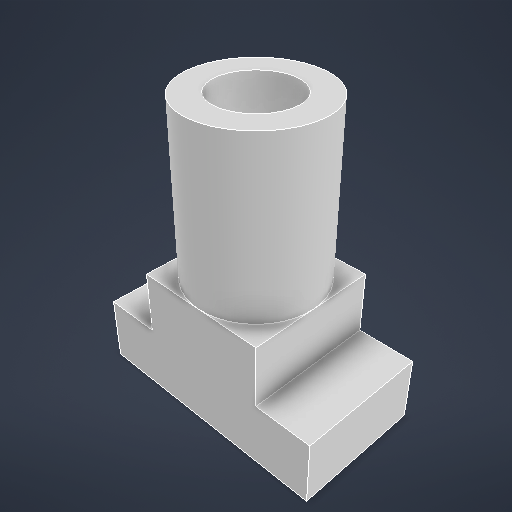
# Autodesk Inventor part: diff_gear_holder_3
Saved by Autodesk Inventor 2025 (Build 290162000, 162)
## iProperties
Created: 2024-07-25
Part Number: diff_gear_holder_3
Material: Generic
Document SubType Name: Modeling
Designer: Garfieldcmix
Density: 1 g/cm^3
Appearance: Default
Author: Garfieldcmix
Autodesk Inventor part; units mm, degrees
ref_plane "YZ Plane" through (0, 0, 0) normal (1, 0, 0) x (0, 1, 0)
ref_plane "XZ Plane" through (0, 0, 0) normal (0, 1, 0) x (-1, 0, 0)
ref_plane "XY Plane" through (0, 0, 0) normal (0, 0, 1) x (1, 0, 0)
sketch "Sketch1" plane through (0, 0, 0) normal (0, 1, 0) x (-1, 0, 0)
  line L0 (0, -8) -> (15, -8)
  line L1 (15, -8) -> (15, 0)
  line L2 (15, 0) -> (0, 0)
  line L3 (0, 0) -> (0, -8)
  line L4 (7.5, 0) -> (7.5, -8) construction
  line L5 (0, -4) -> (15, -4) construction
  line L6 (3.5, 0) -> (3.5, -8)
  line L7 (11.5, -8) -> (11.5, 0)
  circle A0 centre (7.5, -4) radius 2.4
  circle A1 centre (7.5, -4) radius 4
  dimension "d2" = 15
  dimension "d3" = 8
  dimension "d4" = 4
  dimension "d5" = 4
  dimension "d6" = 4.8
  dimension "d7" = 8
  constraints: 16 end point, 5 midpoint, 4 point on line, 3 coincident, 3 perpendicular, 2 centre point, 2 parallel, 1 vertical
  measures "d2" distance of L3.end L0.end
  measures "d3" distance of L2.end L3.end
  measures "d4" distance between parallel lines of L7 L4
  measures "d5" distance between parallel lines of L6 L4
  measures "d6" diameter of A0
  measures "d7" diameter of A1
extrude "Extrusion1" add sketch "Sketch1" along normal blind 4 contours L3 L2 L6 L0 | L7 L2 L1 L0
extrude "Extrusion2" add sketch "Sketch1" along normal blind 7.8 contours L6 A1 L0 | A1 L7 L0 | A1 | L6 L2 A1 | A1 L2 L7
extrude "Extrusion3" add sketch "Sketch1" along normal blind 10.1 from surface at 7.8 contours A1
equation "\"d4\" = 0.5 * d3"
equation "\"d5\" = 0.5 * d3"
body "Solid1"
